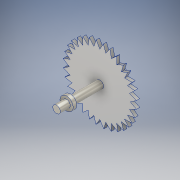
# Autodesk Inventor part: gear
Saved by Autodesk Inventor 2018 (Build 220112000, 112)
## iProperties
Created: 2018-03-07
Part Number: gear
Material: Aluminum 6061
Document SubType Name: Modeling
Designer: kburke4251
Density: 2.7 g/cm^3
Appearance: Aluminum - Flat
Author: kburke4251
Autodesk Inventor part; units mm, degrees
ref_plane "YZ Plane" through (0, 0, 0) normal (1, 0, 0) x (0, 1, 0)
ref_plane "XZ Plane" through (0, 0, 0) normal (0, 1, 0) x (-1, 0, 0)
ref_plane "XY Plane" through (0, 0, 0) normal (0, 0, 1) x (1, 0, 0)
sketch "Sketch1" plane through (0, 0, 0) normal (0, 0, 1) x (1, 0, 0)
  circle A0 centre (0, 0) radius 0.9779
  dimension "d0" = 1.9558
  constraints: 1 centre point, 1 coincident
  measures "d0" diameter of A0
extrude "Extrusion1" add sketch "Sketch1" against normal blind 2.6162
sketch "Sketch2" plane through (0, 0, -2.6162) normal (0, 0, -1) x (-1, 0, 0)
  circle A0 centre (0, 0) radius 1.7272
  dimension "d3" = 3.4544
  constraints: 1 centre point, 1 coincident
  measures "d3" diameter of A0
extrude "Extrusion2" add sketch "Sketch2" along normal blind 0.9652
sketch "Sketch3" plane through (0, 0, -3.5814) normal (0, 0, -1) x (-1, 0, 0)
  circle A0 centre (0, 0) radius 0.9779
  constraints: 1 centre point, 1 coincident
extrude "Extrusion3" add sketch "Sketch3" along normal blind 7.7724
sketch "Sketch4" plane through (0, 0, -11.3538) normal (0, 0, -1) x (-1, 0, 0)
  circle A0 centre (0, 0) radius 8.001
  dimension "d8" = 16.002
  constraints: 1 centre point, 1 coincident
  measures "d8" diameter of A0
extrude "Extrusion4" add sketch "Sketch4" along normal blind 0.8382
sketch "Sketch5" plane through (0, 0, -12.192) normal (0, 0, -1) x (-1, 0, 0)
  circle A0 centre (0, 0) radius 8.001 projected
  circle A1 centre (0, 0) radius 2.5146
  point P0 (-4.9792, 6.2629)
  point P1 (-3.3536, 7.2643)
  point P2 (-1.728, 7.8122)
  point P3 (-0.1024, 8.0003)
  point P4 (1.5232, 7.8547)
  point P5 (5.0214, 6.2291)
  point P6 (6.544, 4.6035)
  point P7 (7.4262, 2.9779)
  point P8 (7.8859, 1.3523)
  point P9 (7.9963, -0.2733)
  point P10 (7.7724, -1.8989)
  point P11 (7.1829, -3.5245)
  point P12 (6.1231, -5.1501)
  point P13 (4.4975, -6.6173)
  point P14 (2.8719, -7.4678)
  point P15 (1.2463, -7.9033)
  point P16 (-0.3793, -7.992)
  point P17 (-2.0049, -7.7457)
  point P18 (-3.6305, -7.1299)
  point P19 (-5.2561, -6.0323)
  point P20 (-6.8817, -4.0814)
  point P21 (-7.6148, -2.4558)
  point P22 (-7.9578, -0.8302)
  point P23 (-7.9614, 0.7954)
  point P24 (-7.6259, 2.421)
  point P25 (-6.9023, 4.0466)
  point P26 (-5.6429, 5.6722)
  point P27 (-3.3816, 7.2513)
  dimension "d11" = 1.6256
  dimension "d12" = 1.6256
  dimension "d13" = 1.6256
  dimension "d14" = 1.6256
  dimension "d15" = 1.6256
  dimension "d16" = 1.6256
  dimension "d17" = 1.6256
  dimension "d18" = 1.6256
  dimension "d19" = 1.6256
  dimension "d20" = 1.6256
  dimension "d21" = 1.6256
  dimension "d22" = 1.6256
  dimension "d23" = 1.6256
  dimension "d24" = 1.6256
  dimension "d25" = 1.6256
  dimension "d26" = 1.6256
  dimension "d27" = 1.6256
  dimension "d28" = 1.6256
  dimension "d29" = 1.6256
  dimension "d30" = 1.6256
  dimension "d32" = 1.6256
  dimension "d33" = 1.6256
  dimension "d34" = 1.6256
  dimension "d35" = 1.6256
  dimension "d36" = 1.6256
  dimension "d37" = 1.6256
  dimension "d39" = 5.0292
  constraints: 1 centre point, 1 coincident, 29 other
  measures "d11" horizontal distance of point (-3.354, 7.264) point (-4.979, 6.263)
  measures "d12" horizontal distance of point (-3.354, 7.264) point (-1.728, 7.812)
  measures "d13" horizontal distance of point (-1.728, 7.812) point (-0.102, 8)
  measures "d14" horizontal distance of point (-0.102, 8) point (1.523, 7.855)
  measures "d15" vertical distance of point (1.523, 7.855) point (5.021, 6.229)
  measures "d16" vertical distance of point (5.021, 6.229) point (6.544, 4.603)
  measures "d17" vertical distance of point (6.544, 4.603) point (7.426, 2.978)
  measures "d18" vertical distance of point (7.426, 2.978) point (7.886, 1.352)
  measures "d19" vertical distance of point (7.886, 1.352) point (7.996, -0.273)
  measures "d20" vertical distance of point (7.996, -0.273) point (7.772, -1.899)
  measures "d21" vertical distance of point (7.772, -1.899) point (7.183, -3.525)
  measures "d22" vertical distance of point (7.183, -3.525) point (6.123, -5.15)
  measures "d23" horizontal distance of point (4.497, -6.617) point (6.123, -5.15)
  measures "d24" horizontal distance of point (4.497, -6.617) point (2.872, -7.468)
  measures "d25" horizontal distance of point (2.872, -7.468) point (1.246, -7.903)
  measures "d26" horizontal distance of point (-0.379, -7.992) point (1.246, -7.903)
  measures "d27" horizontal distance of point (-2.005, -7.746) point (-0.379, -7.992)
  measures "d28" horizontal distance of point (-2.005, -7.746) point (-3.631, -7.13)
  measures "d29" horizontal distance of point (-3.631, -7.13) point (-5.256, -6.032)
  measures "d30" horizontal distance of point (-5.256, -6.032) point (-6.882, -4.081)
  measures "d32" vertical distance of point (-6.882, -4.081) point (-7.615, -2.456)
  measures "d33" vertical distance of point (-7.615, -2.456) point (-7.958, -0.83)
  measures "d34" distance of point (-7.958, -0.83) point (-7.961, 0.795)
  measures "d35" vertical distance of point (-7.961, 0.795) point (-7.626, 2.421)
  measures "d36" vertical distance of point (-7.626, 2.421) point (-6.902, 4.047)
  measures "d37" vertical distance of point (-6.902, 4.047) point (-5.643, 5.672)
  measures "d39" diameter of A1
extrude "Extrusion5" add sketch "Sketch5" along normal blind 2.8448 contours A1
sketch "Sketch6" plane through (0, 0, -15.0368) normal (0, 0, -1) x (-1, 0, 0)
  circle A0 centre (0, 0) radius 0.9779
  dimension "d42" = 1.9558
  constraints: 1 centre point, 1 coincident
  measures "d42" diameter of A0
extrude "Extrusion6" add sketch "Sketch6" along normal blind 2.4892
sketch "Sketch8" plane through (0, 0, -12.192) normal (0, 0, -1) x (-1, 0, 0)
  point P0 (0, 0)
sketch "Sketch9" plane through (0, 0, -12.192) normal (0, 0, -1) x (-1, 0, 0)
  circle A0 centre (0, 0) radius 8.001 projected
  circle A1 centre (0, 0) radius 9.6774
  line L0 (0, 8.001) -> (0.9393, 9.6317)
  line L1 (0.9393, 9.6317) -> (1.5623, 7.847)
  line L2 (1.5623, 7.847) -> (2.7497, 9.2785)
  line L3 (2.7497, 9.2785) -> (3.0623, 7.3918)
  line L4 (3.0623, 7.3918) -> (4.4462, 8.5955)
  line L5 (4.4462, 6.6518) -> (5.9473, 7.6343)
  line L6 (5.9473, 7.6343) -> (5.6517, 5.6634)
  line L7 (5.6517, 5.6634) -> (7.4382, 6.1907)
  line L8 (7.4382, 6.1907) -> (6.494, 4.6738)
  line L9 (6.494, 4.6738) -> (8.4739, 4.6738)
  line L10 (8.4739, 4.6738) -> (7.2714, 3.3381)
  line L11 (7.2714, 3.3381) -> (9.2449, 2.8608)
  line L12 (9.2449, 2.8608) -> (7.7959, 1.8)
  line L13 (7.7959, 1.8) -> (9.6193, 1.0592)
  line L14 (9.6193, 1.0592) -> (8.001, 0)
  line L15 (8.001, 0) -> (9.6193, -1.0592)
  line L16 (9.6193, -1.0592) -> (7.7959, -1.8)
  line L17 (7.7959, -1.8) -> (9.2096, -2.9725)
  line L18 (7.2714, -3.3381) -> (9.2096, -2.9725)
  line L19 (7.2714, -3.3381) -> (8.4739, -4.6738)
  line L20 (8.4739, -4.6738) -> (6.494, -4.6738)
  line L21 (6.494, -4.6738) -> (7.4212, -6.2111)
  line L22 (7.4212, -6.2111) -> (5.6517, -5.6634)
  line L23 (5.6517, -5.6634) -> (6.253, -7.3859)
  line L24 (6.253, -7.3859) -> (4.4462, -6.6518)
  line L25 (4.4462, -6.6518) -> (4.4462, -8.5955)
  line L26 (4.4462, -8.5955) -> (3.0623, -7.3918)
  line L27 (3.0623, -7.3918) -> (2.7497, -9.2785)
  line L28 (2.7497, -9.2785) -> (1.5623, -7.847)
  line L29 (1.5623, -7.847) -> (1.0123, -9.6243)
  line L30 (1.0123, -9.6243) -> (0, -8.001)
  line L31 (0, -8.001) -> (-1.0386, -9.6215)
  line L32 (-1.0386, -9.6215) -> (-1.5623, -7.847)
  line L33 (-1.5623, -7.847) -> (-2.9628, -9.2127)
  line L34 (-2.9628, -9.2127) -> (-3.0623, -7.3918)
  line L35 (-3.0623, -7.3918) -> (-4.7392, -8.4375)
  line L36 (-4.4437, -6.6536) -> (-4.7392, -8.4375)
  line L37 (-4.4437, -6.6536) -> (-6.2508, -7.3878)
  line L38 (-6.2508, -7.3878) -> (-5.6517, -5.6634)
  line L39 (-5.6517, -5.6634) -> (-7.6188, -5.967)
  line L40 (-7.6188, -5.967) -> (-6.494, -4.6738)
  line L41 (-6.494, -4.6738) -> (-8.5183, -4.5924)
  line L42 (-8.5183, -4.5924) -> (-7.2714, -3.3381)
  line L43 (-7.2714, -3.3381) -> (-9.2096, -2.9725)
  line L44 (-9.2096, -2.9725) -> (-7.7959, -1.8)
  line L45 (-7.7959, -1.8) -> (-9.6399, -0.851)
  line L46 (-9.6399, -0.851) -> (-8.001, 0)
  line L47 (-8.001, 0) -> (-9.612, 1.1235)
  line L48 (-9.612, 1.1235) -> (-7.7959, 1.8)
  line L49 (-7.7959, 1.8) -> (-9.1513, 3.1474)
  line L50 (-9.1513, 3.1474) -> (-7.2714, 3.3381)
  line L51 (-8.4739, 4.6738) -> (-7.2714, 3.3381)
  line L52 (-8.4739, 4.6738) -> (-6.494, 4.6738)
  line L53 (-6.494, 4.6738) -> (-7.3128, 6.3383)
  line L54 (-7.3128, 6.3383) -> (-5.6517, 5.6634)
  line L55 (-5.6517, 5.6634) -> (-6.1785, 7.4483)
  line L56 (-6.1785, 7.4483) -> (-4.4437, 6.6536)
  line L57 (-4.4437, 6.6536) -> (-4.4437, 8.5969)
  line L58 (-4.4437, 8.5969) -> (-3.0595, 7.3929)
  line L59 (-3.0595, 7.3929) -> (-2.6348, 9.3118)
  line L60 (-2.6348, 9.3118) -> (-1.5623, 7.847)
  line L61 (-1.5623, 7.847) -> (-0.9432, 9.6313)
  line L62 (0, 8.001) -> (-0.9432, 9.6313)
  line L63 (4.4462, 6.6518) -> (4.4462, 8.5955)
  point P0 (-4.4462, 6.6518)
  dimension "d71" = 19.3548
  constraints: 128 end point, 13 perpendicular, 8 parallel, 1 coincident, 1 vertical, 68 other
extrude "Extrusion7" add sketch "Sketch9" against normal blind 0.8382 contours L15 L16 A0 | A0 L13 L14 | A0 L11 L12 | L17 L18 A0 | A0 L9 L10 | L19 L20 A0 | A0 L7 L8 | L21 L22 A0 | A0 L5 L6 | L23 L24 A0 | A0 L4 L63 | L25 L26 A0 | A0 L2 L3 | L27 L28 A0 | A0 L0 L1 | L29 L30 A0 | A0 L61 L62 | L31 L32 A0 | A0 L59 L60 | L33 L34 A0 | A0 L57 L58 | L35 L36 A0 | A0 L55 L56 | L37 L38 A0 | A0 L53 L54 | L39 L40 A0 | A0 L51 L52 | L41 L42 A0 | A0 L49 L50 | L43 L44 A0 | A0 L47 L48 | L45 L46 A0
body "Solid1"
